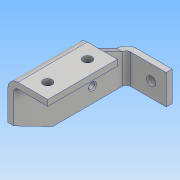
# Autodesk Inventor part: Top_Angle Bracket Small
Saved by Autodesk Inventor 2018.1 (Build 221171000, 171)
## iProperties
Created: 2019-02-12
Part Number: Top_Angle Bracket Small
Material: Aluminum 6061
Document SubType Name: Modeling
Designer: James
Density: 2.7 g/cm^3
Appearance: Aluminum - Flat
Mass: 17.7364 g
Surface Area: 52.0205 cm^2
Volume: 6.56903 cm^3
Author: James
Autodesk Inventor part; units mm, degrees
ref_plane "YZ Plane" through (0, 0, 0) normal (1, 0, 0) x (0, 1, 0)
ref_plane "XZ Plane" through (0, 0, 0) normal (0, 1, 0) x (-1, 0, 0)
ref_plane "XY Plane" through (0, 0, 0) normal (0, 0, 1) x (1, 0, 0)
sketch "Sketch1" plane through (0, 0, 0) normal (0, 1, 0) x (-1, 0, 0)
  line L0 (0, 0) -> (-17, 0)
  line L1 (-17, 0) -> (-17, -3)
  line L2 (-17, -3) -> (0, -3)
  line L3 (0, -3) -> (0, 0)
  line L4 (0, 0) -> (3, 0)
  line L5 (3, 0) -> (3, -20)
  line L6 (3, -20) -> (0, -20)
  line L7 (0, -20) -> (0, 0)
  dimension "d0" = 3
  dimension "d1" = 3
  dimension "d3" = 20
  dimension "d56" = 20
  constraints: 16 end point, 4 parallel, 2 horizontal, 2 perpendicular
  measures "d0" distance of L5.end L6.end
  measures "d1" distance of L0.end L1.end
  measures "d3" distance of L6.end L0.start
  measures "d56" distance between parallel lines of L1 L5
extrude "Extrusion1" add sketch "Sketch1" along normal blind 35
fillet "Fillet1" radius 2 1 edges at (0, 17.5, -3)
fillet "Fillet2" radius 5 1 edges at (-3, 17.5, 0)
sketch "Sketch3" plane through (17, 0, -3) normal (0, 0, -1) x (1, 0, 0)
  line L0 (0, -35) -> (-15, -35) projected
  line L1 (-15, 0) -> (0, 0) projected
  line L2 (0, 0) -> (0, -35) projected
  point P0 (-17, 0)
  point P1 (-7.5, -27.5)
  point P2 (-17, 35)
  point P3 (-17, 0)
  point P4 (-7.5, -7.5)
  point P5 (-17, -35)
  dimension "d21" = 7.5
  dimension "d57" = 7.5
  dimension "d58" = 7.5
  constraints: 1 vertical alignment, 1 other
  measures "d21" distance from line of L2 point (-7.5, -27.5)
  measures "d57" distance from line of L1 point (-7.5, -7.5)
hole "Hole2" at (9.5, 27.5, -3) at (9.5, 7.5, -3) direction (0, 0, 1) diameter 4.5 end through all clearance for "Socket Head Cap Screw" size "M4" standard "Ansi Metric M Profile"
sketch "Sketch4" plane through (-3, 0, -20) normal (-1, 0, 0) x (0, 0, 1)
  line L0 (15, 35) -> (5, 54.5)
  line L1 (5, 54.5) -> (-10, 54.5)
  line L2 (-10, 54.5) -> (-10, 19.5)
  line L3 (0, 0) -> (0, 35) projected
  line L4 (-10, 19.5) -> (0, 0)
  line L5 (5, 54.5) -> (-10, 54.5)
  line L6 (-10, 54.5) -> (-10, 59.5)
  line L7 (-10, 59.5) -> (5, 59.5)
  line L8 (5, 59.5) -> (5, 54.5)
  line L9 (20, 0) -> (20, 35) projected
  line L10 (17, 25.25) -> (17, 29.75) projected
  line L11 (20, 29.75) -> (20, 25.25) projected
  line L12 (17, 25.25) -> (17, 29.75) projected
  line L13 (0, 35) -> (15, 35) projected
  dimension "d30" = 5
  dimension "d32" = 15
  dimension "d34" = 15
  dimension "d59" = 19.5
  constraints: 16 end point, 3 parallel, 2 perpendicular, 1 horizontal
  measures "d30" distance of L0.end L7.end
  measures "d32" distance from line of L9 L7.end
  measures "d34" distance of L6.end L7.end
  measures "d59" vertical distance of L0.start L0.end
extrude "Extrusion2" add sketch "Sketch4" against normal up to surface (3 mm away)
sketch "Sketch5" plane through (-3, 19.5, -30) normal (-1, 0, 0) x (0, 0, 1)
  line L0 (10, -19.5) -> (25, -19.5) projected
  line L1 (0, 40) -> (0, 0) projected
  line L2 (15, 40) -> (0, 40)
  line L3 (0, 40) -> (0, 37)
  line L4 (0, 37) -> (15, 37)
  line L5 (15, 37) -> (15, 40)
  line L6 (25, 15.5) -> (15, 35) projected
  line L7 (15, 35) -> (15, 40) projected
  line L8 (15, 40) -> (0, 40) projected
  line L9 (0, 40) -> (0, 0) projected
  line L10 (0, 0) -> (10, -19.5) projected
  line L11 (25, 15.5) -> (25, -19.5) projected
  point P0 (30, -19.5)
  dimension "d52" = 3
  dimension "d53" = 15
  constraints: 8 end point, 2 parallel, 1 horizontal, 1 perpendicular, 1 point on line
  measures "d52" distance of L1.start L3.end
  measures "d53" distance of L2.start L1.start
extrude "Extrusion3" add sketch "Sketch5" against normal blind 23 contours L1 L2 L5 L4
fillet "Fillet3" radius 2 1 edges at (0, 56.5, -22.5)
fillet "Fillet4" radius 5 1 edges at (-3, 59.5, -22.5)
sketch "Sketch6" plane through (22, 59.5, -15) normal (0, 1, 0) x (-1, 0, 0)
  line L0 (2, -15) -> (2, 0) projected
  point P0 (9.5, -7.5)
  point P1 (2, -7.5)
  point P2 (2, -7.5)
  dimension "d54" = 7.5
  constraints: 2 horizontal alignment, 1 midpoint
  measures "d54" distance from line of point (9.5, -7.5) L0
hole "Hole3" at (12.5, 59.5, -22.5) direction (0, -1, 0) diameter 4.5 end through all clearance for "Flat Head Machine Screw" size "M4" standard "Ansi Metric M Profile"
sketch "Sketch7" plane through (-3, 0, -20) normal (-1, 0, 0) x (0, 0, 1)
  line L0 (-10, 54.5) -> (5, 54.5) projected
  line L1 (-10, 54.5) -> (-10, 19.5) projected
  point P0 (20, 0)
  point P1 (-2.5, 39.5)
  dimension "d60" = 15
  dimension "d61" = 7.5
  measures "d60" distance from line of point (-2.5, 39.5) L0
  measures "d61" distance from line of point (-2.5, 39.5) L1
hole "Hole4" at (-3, 39.5, -22.5) direction (1, 0, 0) diameter 3 end through all
chamfer "Chamfer1" distance 0.5 angle 45 2 edges at (-3, 39.5, -24) (0, 39.5, -24)
equation "\"d1\" = d0"
equation "\"d21\" = d19"
equation "\"d58\" = d57"
equation "\"d19\" = 7.5"
body "Solid1"
